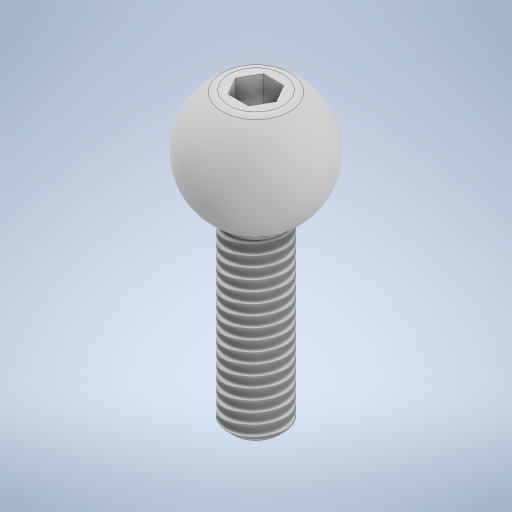
# Autodesk Inventor part: Pillow Ball
Saved by Autodesk Inventor 2024 (Build 280153000, 153)
## iProperties
Created: 2023-07-03
Part Number: Pillow Ball
Material: Generic
Document SubType Name: Modeling
Designer: patel
Density: 1 g/cm^3
Appearance: Default
Author: patel
Autodesk Inventor part; units mm, degrees
ref_plane "YZ Plane" through (0, 0, 0) normal (1, 0, 0) x (0, 1, 0)
ref_plane "XY Plane" through (0, 0, 0) normal (0, 0, 1) x (1, 0, 0)
sketch "Sketch1" plane through (0, 0, 0) normal (0, 0, 1) x (1, 0, 0)
  line L0 (0, 9.0251) -> (0, -20.025) projected
  arc A0 (0, 4.1275) -> (-1.905, -3.6616) centre (0, 0) ccw
  line L1 (-1.905, -3.6616) -> (-1.905, -15.875)
  line L2 (-1.905, -15.875) -> (0, -15.875)
  dimension "d0" = 8.255
  dimension "d1" = 15.875
  dimension "d2" = 3.81
  constraints: 4 end point, 2 point on circle, 2 point on line, 1 centre point, 1 coincident, 1 perpendicular, 1 vertical
  measures "d0" diameter of A0
  measures "d1" distance from line of L2 point (0, 0)
  measures "d2" diameter of L1 L0
revolve "Revolution1" add sketch "Sketch1" angle 360 about axis through (0, 0, 0) along (0, -1, 0)
fillet "Fillet1" radius 0.381 1 edges at (1.905, -3.6616, 0)
chamfer "Chamfer1" distance 0.381 angle 45 1 edges at (1.905, -15.875, 0)
sketch "Sketch2" plane through (0, 0, 0) normal (0, 0, 1) x (1, 0, 0)
  line L0 (-1.524, -15.875) -> (-1.905, -15.494) projected
  line L1 (-1.905, -15.494) -> (-1.905, -3.886) projected
  arc A0 (-1.905, -3.886) -> (-2.0928, -3.5576) centre (-2.286, -3.886) ccw projected
  arc A1 (2.0928, -3.5576) -> (-2.0928, -3.5576) centre (0, 0) ccw projected
  arc A2 (2.0928, -3.5576) -> (1.905, -3.886) centre (2.286, -3.886) ccw projected
  line L2 (1.905, -3.886) -> (1.905, -15.494) projected
  line L3 (1.905, -15.494) -> (1.524, -15.875) projected
  line L4 (1.524, -15.875) -> (-1.524, -15.875) projected
  point P0 (2.0638, 3.5745)
  constraints: 1 point on circle
ref_plane "Work Plane1" through (0, 0, 0) normal (0, 1, 0) x (-1, 0, 0)
ref_plane "Work Plane2" through (2.0638, 3.5745, 0) normal (0, 1, 0) x (-1, 0, 0)
split "Split1" plane through (2.0638, 3.5745, 0) removes the side toward (0, 1, 0)
fillet "Fillet2" radius 0.8128 1 edges at (2.0638, 3.5745, 0)
sketch "Sketch3" plane through (0, 3.5745, 0) normal (0, 1, 0) x (1, 0, 0)
  circle A0 centre (0, 0) radius 1.524 projected
  line L0 (1.3748, 0) -> (0.6874, -1.1906)
  line L1 (0.6874, -1.1906) -> (-0.6874, -1.1906)
  line L2 (-0.6874, -1.1906) -> (-1.3748, 0)
  line L3 (-1.3748, 0) -> (-0.6874, 1.1906)
  line L4 (-0.6874, 1.1906) -> (0.6874, 1.1906)
  line L5 (0.6874, 1.1906) -> (1.3748, 0)
  dimension "d11" = 2.3813
  constraints: 12 end point, 1 coincident, 1 horizontal, 13 other
  measures "d11" distance between parallel lines of L1 L4
extrude "Extrusion1" cut sketch "Sketch3" against normal blind 2.54 contours L0 L1 L2 L3 L4 L5
thread "Thread1" size "8-36 UNF" class "2A" standard "ANSI Unified Screw Threads" full length
body "Solid1"
